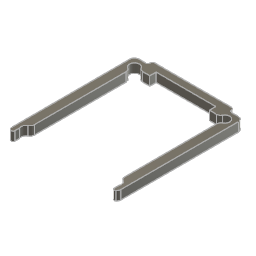
Assy v13 (Autodesk Fusion 360 archive; units mm, degrees)
design "Screen Spacer"
Autodesk Fusion 360 part; units mm, degrees
sketch "Sketch1" plane through (0, 0, 0) normal (0, 1, 0) x (1, 0, 0)
  line L0 (0, 0) -> (20, 0) construction
  line L1 (20, 0) -> (20, 24) construction
  line L2 (20, 24) -> (0, 24) construction
  line L3 (0, 24) -> (0, 0) construction
  circle A0 centre (0, 24) radius 1.1
  circle A1 centre (20, 24) radius 1.1
  circle A2 centre (20, 0) radius 1.1
  circle A3 centre (0, 0) radius 1.1
  line L4 (-2, 26) -> (22, 26)
  line L5 (22, 26) -> (22, -2)
  line L6 (22, -2) -> (-2, -2)
  line L7 (-2, -2) -> (-2, 26)
  line L8 (0, 24) -> (20, 24)
  line L9 (20, 24) -> (20, 0)
  line L10 (20, 0) -> (0, 0)
  line L11 (0, 0) -> (0, 24)
  dimension "d1" = 24
  dimension "d2" = 20
  dimension "d3" = 2.2
  dimension "d4" = 2
  dimension "d5" = 2
  dimension "d6" = 2
  dimension "d7" = 2
  constraint horizontal L0
  constraint vertical L1
  constraint horizontal L2
  constraint vertical L3
  constraint coincident L0.start L3.end
  constraint coincident L2.end L3.start
  constraint coincident L1.end L2.start
  constraint coincident L0.end L1.start
  constraint equal A0 A3
  constraint equal A0 A1
  constraint equal A1 A2
  constraint horizontal L4
  constraint vertical L5
  constraint horizontal L6
  constraint vertical L7
  constraint horizontal L8
  constraint vertical L9
  constraint horizontal L10
  constraint vertical L11
  measures "d1" distance of L0.start L2.end
  measures "d2" distance of L1.end L2.end
  measures "d3" diameter of A0
  measures "d4" distance of L2 L4
  measures "d5" distance of L1 L5
  measures "d6" distance of L0 L6
  measures "d7" distance of L3 L7
extrude "Extrude1" add sketch "Sketch1" along normal blind 2
fillet "Fillet1" radius 1 8 edges at (1.1, 1, -24) (0, 1, -22.9) (0, 1, -1.1) (18.9, 1, -24) (1.1, 1, 0) (20, 1, -22.9) (20, 1, -1.1) (18.9, 1, 0)
fillet "Fillet2" radius 1 4 edges at (-2, 1, -26) (-2, 1, 2) (22, 1, 2) (22, 1, -26)
extrude "Extrude2" cut 1 faces at (13.6667, 0.6667, 2) along direction (0, 0, -1) up to surface (2 mm away)
fillet "Fillet3" radius 0.4 2 edges at (-1, 1, 2) (21, 1, 2)
sketch "Sketch2" plane through (0, 2, 0) normal (0, 1, 0) x (-1, 0, 0)
  arc A0 (-21, 1.4472) -> (-21.6667, 1.7454) centre (-21.4, 1.4472) ccw
  arc A1 (-21.6667, 1.7454) -> (-22, 1) centre (-21, 1) ccw
  line L0 (-22, 1) -> (-22, -25)
  arc A2 (-22, -25) -> (-21, -26) centre (-21, -25) ccw
  line L1 (-21, -26) -> (1, -26)
  arc A3 (1, -26) -> (2, -25) centre (1, -25) ccw
  line L2 (2, -25) -> (2, 1)
  arc A4 (2, 1) -> (1.6667, 1.7454) centre (1, 1) ccw
  arc A5 (1.6667, 1.7454) -> (1, 1.4472) centre (1.4, 1.4472) ccw
  line L3 (1, 1.4472) -> (1, 0.4583)
  arc A6 (0.5238, -0.9673) -> (1, 0.4583) centre (0, 0) ccw
  arc A7 (0.5238, -0.9673) -> (0, -1.8466) centre (1, -1.8466) ccw
  line L4 (0, -1.8466) -> (0, -22.1534)
  arc A8 (0, -22.1534) -> (0.5238, -23.0327) centre (1, -22.1534) ccw
  arc A9 (-0.9673, -24.5238) -> (0.5238, -23.0327) centre (0, -24) ccw
  arc A10 (-0.9673, -24.5238) -> (-1.8466, -24) centre (-1.8466, -25) ccw
  line L5 (-1.8466, -24) -> (-18.1534, -24)
  arc A11 (-18.1534, -24) -> (-19.0327, -24.5238) centre (-18.1534, -25) ccw
  arc A12 (-20.5238, -23.0327) -> (-19.0327, -24.5238) centre (-20, -24) ccw
  arc A13 (-20.5238, -23.0327) -> (-20, -22.1534) centre (-21, -22.1534) ccw
  line L6 (-20, -22.1534) -> (-20, -1.8466)
  arc A14 (-20, -1.8466) -> (-20.5238, -0.9673) centre (-21, -1.8466) ccw
  arc A15 (-21, 0.4583) -> (-20.5238, -0.9673) centre (-20, 0) ccw
  line L7 (-21, 0.4583) -> (-21, 1.4472)
  line L8 (-3.4, -24) -> (-16.6, -24)
  line L9 (-16.6, -24) -> (-16.6, -25.4)
  line L10 (-16.6, -25.4) -> (-3.4, -25.4)
  line L11 (-3.4, -25.4) -> (-3.4, -24)
  line L12 (-1, -26) -> (-1, -27)
  line L13 (-1, -27) -> (-19, -27)
  line L14 (-19, -27) -> (-19, -26)
  line L15 (-1, -26) -> (-19, -26)
  dimension "d18" = 1.4
  dimension "d19" = 13.2
  dimension "d20" = 1
  dimension "d21" = 18
  constraint horizontal L8
  constraint vertical L9
  constraint horizontal L10
  constraint vertical L11
  constraint coincident L5 L8.start
  constraint midpoint L5 L8
  constraint coincident L1 L12.start
  constraint perpendicular L1 L12
  constraint perpendicular L12 L13
  constraint coincident L1 L14.end
  constraint perpendicular L1 L14
  constraint midpoint L1 L15
  measures "d18" distance of L8.end L9.end
  measures "d19" distance of L9.end L10.end
  measures "d20" distance of L12.start L12.end
  measures "d21" distance of L12.end L13.end
extrude "Extrude3" cut sketch "Sketch2" against normal up to surface (2 mm away) contours L5 L8 L9 L10 L11
extrude "Extrude4" add sketch "Sketch2" against normal up to surface (2 mm away) contours L1 L12 L13 L14 L15
fillet "Fillet5" radius 0.5 4 edges at (1, 1, -26) (1, 1, -27) (19, 1, -27) (19, 1, -26)

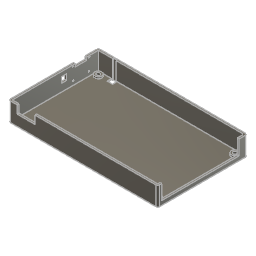
design "Main Case"
Autodesk Fusion 360 part; units mm, degrees
sketch "Sketch1" plane through (0, 0, 0) normal (0, 1, 0) x (1, 0, 0)
  line L0 (0, 0) -> (162, 0) construction
  line L1 (162, 0) -> (162, 95) construction
  line L2 (162, 95) -> (0, 95) construction
  line L3 (0, 95) -> (0, 0) construction
  line L4 (4, 91) -> (158, 91) construction
  line L5 (158, 91) -> (158, 4) construction
  line L6 (158, 4) -> (4, 4) construction
  line L7 (4, 4) -> (4, 91) construction
  circle A0 centre (4, 91) radius 2
  circle A1 centre (4, 4) radius 2
  circle A2 centre (158, 4) radius 2
  circle A3 centre (158, 91) radius 2
  line L8 (-1, 96) -> (163, 96)
  line L9 (163, 96) -> (163, -1)
  line L10 (163, -1) -> (-1, -1)
  line L11 (-1, -1) -> (-1, 96)
  line L12 (4, 91) -> (158, 4) construction
  line L13 (162, 95) -> (0, 0) construction
  dimension "d1" = 162
  dimension "d2" = 95
  dimension "d7" = 4
  dimension "d8" = 1
  dimension "d9" = 1
  dimension "d10" = 1
  dimension "d11" = 1
  dimension "d35" = 87
  dimension "d36" = 154
  constraint horizontal L0
  constraint vertical L1
  constraint horizontal L2
  constraint vertical L3
  constraint coincident L0.start L3.end
  constraint horizontal L4
  constraint vertical L5
  constraint horizontal L6
  constraint vertical L7
  constraint coincident L4.start L7.end
  constraint coincident L6.end L7.start
  constraint coincident L5.end L6.start
  constraint coincident L4.end L5.start
  constraint equal A0 A1
  constraint equal A1 A2
  constraint equal A2 A3
  constraint horizontal L8
  constraint vertical L9
  constraint horizontal L10
  constraint vertical L11
  constraint midpoint L12 L13
  measures "d1" distance of L1.end L2.end
  measures "d2" distance of L0.start L2.end
  measures "d7" diameter of A0
  measures "d8" distance of L2 L8
  measures "d9" distance of L1 L9
  measures "d10" distance of L0 L10
  measures "d11" distance of L3 L11
  measures "d35" distance of L4.start L6.end
  measures "d36" distance of L4.start L4.end
extrude "Extrude1" add sketch "Sketch1" along normal blind 1.2
sketch "Sketch2" plane through (0, 1.2, 0) normal (0, 1, 0) x (-1, 0, 0)
  circle A0 centre (-4, -91) radius 2
  circle A1 centre (-158, -4) radius 2
  circle A2 centre (-4, -4) radius 2
  circle A3 centre (-158, -91) radius 2
  line L0 (1, 1) -> (-163, 1)
  line L1 (-163, 1) -> (-163, -96)
  line L2 (-163, -96) -> (1, -96)
  line L3 (1, -96) -> (1, 1)
  circle A4 centre (-4, -91) radius 4
  circle A5 centre (-158, -91) radius 4
  circle A6 centre (-158, -4) radius 4
  circle A7 centre (-4, -4) radius 4
  dimension "d23" = 8
  constraint concentric A0 A4
  constraint concentric A3 A5
  constraint concentric A1 A6
  constraint concentric A2 A7
  constraint equal A4 A7
  constraint equal A4 A5
  constraint equal A5 A6
  measures "d23" diameter of A4
extrude "Extrude2" add sketch "Sketch2" along normal blind 2 contours A4 | A5 | A6 | A7
sketch "Sketch3" plane through (0, 0, 0) normal (0, -1, 0) x (1, 0, 0)
  circle A0 centre (4, -91) radius 2
  circle A1 centre (158, -4) radius 2
  circle A2 centre (4, -4) radius 2
  circle A3 centre (158, -91) radius 2
  line L0 (163, 1) -> (-1, 1)
  line L1 (-1, 1) -> (-1, -96)
  line L2 (-1, -96) -> (163, -96)
  line L3 (163, -96) -> (163, 1)
  line L4 (-1, 1) -> (163, 1)
  line L5 (163, 1) -> (163, -96)
  line L6 (163, -96) -> (-1, -96)
  line L7 (-1, -96) -> (-1, 1)
  line L8 (-3, 3) -> (165, 3)
  line L9 (165, 3) -> (165, -98)
  line L10 (165, -98) -> (-3, -98)
  line L11 (-3, -98) -> (-3, 3)
  dimension "d17" = 2
  dimension "d18" = 2
  dimension "d19" = 2
  dimension "d20" = 2
  constraint horizontal L4
  constraint vertical L5
  constraint horizontal L6
  constraint vertical L7
  constraint coincident L2.end L3.start
  constraint coincident L0.end L1.start
  constraint horizontal L8
  constraint vertical L9
  constraint horizontal L10
  constraint vertical L11
  measures "d17" distance of L4 L8
  measures "d18" distance of L7 L11
  measures "d19" distance of L6 L10
  measures "d20" distance of L5 L9
extrude "Extrude3" add sketch "Sketch3" against normal blind 21.3 contours L8 L9 L10 L11
fillet "Fillet1" radius 2 4 edges at (-3, 10.65, -98) (-3, 10.65, 3) (165, 10.65, 3) (165, 10.65, -98)
sketch "Sketch4" plane through (0, 1.2, 0) normal (0, 1, 0) x (-1, 0, 0)
  circle A0 centre (-4, -4) radius 4
  circle A1 centre (-4, -91) radius 4
  circle A2 centre (-158, -4) radius 4
  circle A3 centre (-158, -91) radius 4
  line L0 (1, 1) -> (-163, 1)
  line L1 (-163, 1) -> (-163, -96)
  line L2 (-163, -96) -> (1, -96)
  line L3 (1, -96) -> (1, 1)
  line L4 (-14, -96) -> (-20, -96)
  line L5 (-20, -96) -> (-20, -91)
  line L6 (-20, -91) -> (-14, -91)
  line L7 (-14, -91) -> (-14, -96)
  dimension "d30" = 6
  dimension "d31" = 5
  dimension "d32" = 15
  constraint horizontal L4
  constraint vertical L5
  constraint horizontal L6
  constraint vertical L7
  constraint coincident L2 L4.end
  measures "d30" distance of L4.start L4.end
  measures "d31" distance of L4.end L5.end
  measures "d32" distance of L2.end L4.start
extrude "Extrude4" cut sketch "Sketch4" against normal up to surface (1.2 mm away) contours L2 L4 L5 L6 L7
sketch "Sketch5" plane through (0, 21.3, 0) normal (0, 1, 0) x (-1, 0, 0)
  arc A0 (-165, -96) -> (-163, -98) centre (-163, -96) ccw
  line L0 (-163, -98) -> (1, -98)
  arc A1 (1, -98) -> (3, -96) centre (1, -96) ccw
  line L1 (3, -96) -> (3, 1)
  arc A2 (3, 1) -> (1, 3) centre (1, 1) ccw
  line L2 (1, 3) -> (-163, 3)
  arc A3 (-163, 3) -> (-165, 1) centre (-163, 1) ccw
  line L3 (-165, 1) -> (-165, -96)
  line L4 (1, -96) -> (-163, -96)
  line L5 (-163, -96) -> (-163, 1)
  line L6 (-163, 1) -> (1, 1)
  line L7 (1, 1) -> (1, -96)
  line L8 (-15, -96) -> (-19, -96)
  line L9 (-19, -96) -> (-19, -96.8)
  line L10 (-19, -96.8) -> (-15, -96.8)
  line L11 (-15, -96.8) -> (-15, -96)
  point P0 (-14, -96)
  dimension "d37" = 4
  dimension "d38" = 1
  dimension "d39" = 0.8
  constraint horizontal L8
  constraint vertical L9
  constraint horizontal L10
  constraint vertical L11
  constraint coincident L4 L8.start
  measures "d37" distance of L9.end L10.end
  measures "d38" distance of L8.start P0
  measures "d39" distance of L8.end L9.end
extrude "Extrude5" cut sketch "Sketch5" against normal up to surface (21.3 mm away) contours L4 L8 L9 L10 L11
sketch "Sketch6" plane through (165, 0, 0) normal (1, 0, 0) x (0, 0, -1)
  line L0 (96, 0) -> (96, 21.3)
  line L1 (96, 21.3) -> (-1, 21.3)
  line L2 (-1, 21.3) -> (-1, 0)
  line L3 (-1, 0) -> (96, 0)
  line L4 (1.7, 21.3) -> (88.7, 21.3)
  line L5 (88.7, 21.3) -> (88.7, 4.8)
  line L6 (88.7, 4.8) -> (1.7, 4.8)
  line L7 (1.7, 4.8) -> (1.7, 21.3)
  dimension "d42" = 2.7
  dimension "d43" = 87
  dimension "d44" = 4.8
  constraint horizontal L4
  constraint vertical L5
  constraint horizontal L6
  constraint vertical L7
  constraint coincident L1 L4.end
  measures "d42" distance of L2 L7
  measures "d43" distance of L4.start L4.end
  measures "d44" distance of L3 L5.end
extrude "Extrude6" cut sketch "Sketch6" against normal up to surface (2 mm away) contours L1 L4 L5 L6 L7
sketch "Sketch7" plane through (-3, 0, 0) normal (-1, 0, 0) x (0, 0, 1)
  line L0 (1, 0) -> (1, 21.3)
  line L1 (1, 21.3) -> (-96, 21.3)
  line L2 (-96, 21.3) -> (-96, 0) construction
  line L3 (-96, 0) -> (1, 0)
  line L4 (-85.5, 20) -> (-67.5, 20) construction
  line L5 (-67.5, 20) -> (-67.5, 6) construction
  line L6 (-67.5, 6) -> (-85.5, 6) construction
  line L7 (-85.5, 6) -> (-85.5, 20) construction
  line L8 (-83, 21.3) -> (-70, 21.3) construction
  line L9 (-70, 21.3) -> (-70, 18.7) construction
  line L10 (-70, 18.7) -> (-83, 18.7) construction
  line L11 (-83, 18.7) -> (-83, 21.3) construction
  line L12 (-83, 21.3) -> (-70, 18.7) construction
  circle A0 centre (-85.5, 20) radius 0.9
  circle A1 centre (-85.5, 6) radius 0.9
  circle A2 centre (-67.5, 6) radius 0.9
  circle A3 centre (-67.5, 20) radius 0.9
  dimension "d47" = 14
  dimension "d48" = 18
  dimension "d51" = 13
  dimension "d52" = 2.6
  dimension "d53" = 26
  dimension "d54" = 1.8
  constraint horizontal L4
  constraint vertical L5
  constraint horizontal L6
  constraint vertical L7
  constraint horizontal L8
  constraint vertical L9
  constraint horizontal L10
  constraint vertical L11
  constraint midpoint L4 L12
  constraint coincident L1 L8.end
  constraint coincident L4.start L7.end
  constraint coincident L6.end L7.start
  constraint coincident L5.end L6.start
  constraint coincident L4.end L5.start
  constraint equal A2 A3
  constraint equal A1 A2
  constraint equal A0 A1
  measures "d47" distance of L4.end L5.end
  measures "d48" distance of L4.start L4.end
  measures "d51" distance of L8.start L8.end
  measures "d52" distance of L8.start L10.end
  measures "d53" distance of L1.end L8.end
  measures "d54" diameter of A0
extrude "Extrude7" cut sketch "Sketch7" against normal up to surface (2 mm away)
sketch "Sketch8" plane through (-3, 0, 0) normal (-1, 0, 0) x (0, 0, 1)
  circle A0 centre (-67.5, 6) radius 0.9
  circle A1 centre (-85.5, 6) radius 0.9
  line L0 (1, 0) -> (1, 21.3)
  line L1 (1, 21.3) -> (-96, 21.3)
  line L2 (-96, 21.3) -> (-96, 0)
  line L3 (-96, 0) -> (1, 0)
  line L4 (-83, 21.3) -> (-70, 21.3)
  line L5 (-70, 21.3) -> (-70, 18.1)
  line L6 (-70, 18.1) -> (-83, 18.1)
  line L7 (-83, 18.1) -> (-83, 21.3)
  point P0 (-83, 21.3)
  point P1 (-70, 21.3)
  dimension "d59" = 3.2
  constraint horizontal L4
  constraint vertical L5
  constraint horizontal L6
  constraint vertical L7
  constraint coincident P0 L4.start
  constraint coincident L5 P1
  measures "d59" distance of P0 L6.end
extrude "Extrude8" cut sketch "Sketch8" against normal up to surface (2 mm away) contours L1 L4 L5 L6 L7
sketch "Sketch9" plane through (-3, 0, 0) normal (-1, 0, 0) x (0, 0, 1)
  line L0 (-83, 18.1) -> (-83, 21.3)
  line L1 (-83, 21.3) -> (-96, 21.3)
  line L2 (-96, 21.3) -> (-96, 0)
  line L3 (-96, 0) -> (1, 0)
  line L4 (1, 0) -> (1, 21.3)
  line L5 (1, 21.3) -> (-70, 21.3)
  line L6 (-70, 21.3) -> (-70, 18.1)
  line L7 (-70, 18.1) -> (-83, 18.1)
  circle A0 centre (-67.5, 20) radius 0.9
  circle A1 centre (-67.5, 6) radius 0.9
  circle A2 centre (-85.5, 20) radius 0.9
  circle A3 centre (-85.5, 6) radius 0.9
  line L8 (-60.2, 16.2) -> (-54.8, 16.2)
  line L9 (-54.8, 16.2) -> (-54.8, 9.8)
  line L10 (-54.8, 9.8) -> (-60.2, 9.8)
  line L11 (-60.2, 9.8) -> (-60.2, 16.2)
  line L12 (-67.5, 20) -> (-67.5, 6) construction
  line L13 (-67.5, 6) -> (-57.5, 13) construction
  line L14 (-57.5, 13) -> (-67.5, 20) construction
  line L15 (-60.2, 16.2) -> (-54.8, 9.8) construction
  dimension "d60" = 6.4
  dimension "d61" = 5.4
  dimension "d62" = 10
  constraint horizontal L8
  constraint vertical L9
  constraint horizontal L10
  constraint vertical L11
  constraint coincident A0.centre L12.start
  constraint coincident A1.centre L12.end
  constraint equal L13 L14
  constraint midpoint L13.end L15
  measures "d60" distance of L8.end L9.end
  measures "d61" distance of L8.start L8.end
  measures "d62" distance of L12 L13.end
extrude "Extrude9" cut sketch "Sketch9" against normal up to surface (2 mm away) contours L8 L9 L10 L11
sketch "Sketch10" plane through (0, 0, 3) normal (0, 0, 1) x (1, 0, 0)
  line L0 (163, 0) -> (163, 21.3)
  line L1 (163, 21.3) -> (-1, 21.3)
  line L2 (-1, 21.3) -> (-1, 0)
  line L3 (-1, 0) -> (163, 0)
  line L4 (6.5, 22.2) -> (26.5, 22.2)
  line L5 (26.5, 22.2) -> (26.5, 12.2)
  line L6 (26.5, 12.2) -> (6.5, 12.2)
  line L7 (6.5, 12.2) -> (6.5, 22.2)
  line L8 (6.5, 22.2) -> (26.5, 12.2) construction
  point P0 (16.5, 17.2)
  dimension "d66" = 20
  dimension "d67" = 10
  dimension "d68" = 17.2
  dimension "d69" = 17.5
  constraint horizontal L4
  constraint vertical L5
  constraint horizontal L6
  constraint vertical L7
  constraint midpoint L8 P0
  measures "d66" distance of L4.start L4.end
  measures "d67" distance of L4.end L5.end
  measures "d68" vertical distance of L2.end P0
  measures "d69" horizontal distance of L1.end P0
extrude "Extrude10" cut sketch "Sketch10" against normal up to surface (2 mm away) contours L1 L5 L6 L7
equation "d21 = -20.00 mm - 1.3 mm"
equation "d42 = 1.7 mm + 1 mm"
equation "d44 = 3.2 mm + 1.6 mm"
equation "d68 = 1.6 mm + 15.6 mm"

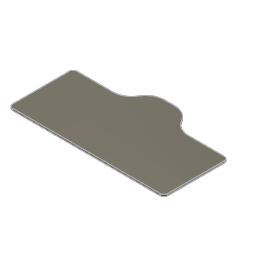
design "Culture Retainer Wall"
Autodesk Fusion 360 part; units mm, degrees
sketch "Sketch1" plane through (0, 0, 0) normal (0, 1, 0) x (1, 0, 0)
  line L0 (0, 0) -> (82, 0)
  line L1 (82, 0) -> (82, 34)
  line L2 (82, 34) -> (0, 34)
  line L3 (0, 34) -> (0, 0)
  line L4 (31, 44) -> (51, 44)
  line L5 (51, 44) -> (51, 34)
  line L6 (51, 34) -> (31, 34)
  line L7 (31, 34) -> (31, 44)
  dimension "d1" = 82
  dimension "d2" = 34
  dimension "d3" = 20
  dimension "d4" = 10
  constraint horizontal L0
  constraint vertical L1
  constraint horizontal L2
  constraint vertical L3
  constraint coincident L0.start L3.end
  constraint horizontal L4
  constraint vertical L5
  constraint horizontal L6
  constraint vertical L7
  constraint midpoint L2 L6
  measures "d1" distance of L1.end L2.end
  measures "d2" distance of L0.start L2.end
  measures "d3" distance of L4.start L4.end
  measures "d4" distance of L4.end L5.end
extrude "Extrude1" add sketch "Sketch1" along normal blind 1
fillet "Fillet1" radius 10 4 edges at (51, 0.5, -34) (51, 0.5, -44) (31, 0.5, -44) (31, 0.5, -34)
fillet "Fillet2" radius 2 4 edges at (0, 0.5, 0) (82, 0.5, 0) (82, 0.5, -34) (0, 0.5, -34)

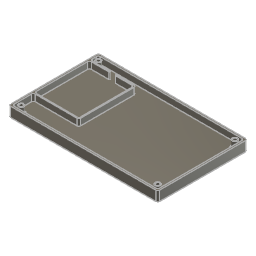
design "Bottom Case (Battery Tray)"
Autodesk Fusion 360 part; units mm, degrees
sketch "Sketch1" plane through (0, 0, 0) normal (0, 1, 0) x (1, 0, 0)
  line L0 (0, 0) -> (162, 0) construction
  line L1 (162, 0) -> (162, 95) construction
  line L2 (162, 95) -> (0, 95) construction
  line L3 (0, 95) -> (0, 0) construction
  line L4 (4, 91) -> (158, 91) construction
  line L5 (158, 91) -> (158, 4) construction
  line L6 (158, 4) -> (4, 4) construction
  line L7 (4, 4) -> (4, 91) construction
  circle A0 centre (4, 91) radius 2
  circle A1 centre (4, 4) radius 2
  circle A2 centre (158, 4) radius 2
  circle A3 centre (158, 91) radius 2
  line L8 (-1, 96) -> (163, 96)
  line L9 (163, 96) -> (163, -1)
  line L10 (163, -1) -> (-1, -1)
  line L11 (-1, -1) -> (-1, 96)
  line L12 (4, 91) -> (158, 4) construction
  line L13 (162, 95) -> (0, 0) construction
  dimension "d1" = 162
  dimension "d2" = 95
  dimension "d7" = 4
  dimension "d8" = 1
  dimension "d9" = 1
  dimension "d10" = 1
  dimension "d11" = 1
  dimension "d55" = 87
  dimension "d56" = 154
  constraint horizontal L0
  constraint vertical L1
  constraint horizontal L2
  constraint vertical L3
  constraint coincident L0.start L3.end
  constraint horizontal L4
  constraint vertical L5
  constraint horizontal L6
  constraint vertical L7
  constraint coincident L4.start L7.end
  constraint coincident L6.end L7.start
  constraint coincident L5.end L6.start
  constraint coincident L4.end L5.start
  constraint equal A0 A1
  constraint equal A1 A2
  constraint equal A2 A3
  constraint horizontal L8
  constraint vertical L9
  constraint horizontal L10
  constraint vertical L11
  constraint midpoint L12 L13
  measures "d1" distance of L1.end L2.end
  measures "d2" distance of L0.start L2.end
  measures "d7" diameter of A0
  measures "d8" distance of L2 L8
  measures "d9" distance of L3 L11
  measures "d10" distance of L0 L10
  measures "d11" distance of L1 L9
  measures "d55" distance of L4.start L6.end
  measures "d56" distance of L4.start L4.end
extrude "Extrude1" add sketch "Sketch1" along normal blind 3
sketch "Sketch2" plane through (0, 0, 0) normal (0, -1, 0) x (1, 0, 0)
  circle A0 centre (4, -91) radius 2
  circle A1 centre (158, -4) radius 2
  circle A2 centre (4, -4) radius 2
  circle A3 centre (158, -91) radius 2
  line L0 (163, 1) -> (-1, 1)
  line L1 (-1, 1) -> (-1, -96)
  line L2 (-1, -96) -> (163, -96)
  line L3 (163, -96) -> (163, 1)
  line L4 (-3, 3) -> (165, 3)
  line L5 (165, 3) -> (165, -98)
  line L6 (165, -98) -> (-3, -98)
  line L7 (-3, -98) -> (-3, 3)
  dimension "d16" = 2
  dimension "d17" = 2
  dimension "d18" = 2
  dimension "d19" = 2
  constraint horizontal L4
  constraint vertical L5
  constraint horizontal L6
  constraint vertical L7
  measures "d16" distance of L0 L4
  measures "d17" distance of L2 L6
  measures "d18" distance of L1 L7
  measures "d19" distance of L3 L5
extrude "Extrude2" add sketch "Sketch2" against normal blind 9 contours L4 L5 L6 L7
fillet "Fillet2" radius 2 4 edges at (-3, 4.5, 3) (-3, 4.5, -98) (165, 4.5, -98) (165, 4.5, 3)
sketch "Sketch3" plane through (0, 3, 0) normal (0, 1, 0) x (-1, 0, 0)
  circle A0 centre (-4, -91) radius 2
  circle A1 centre (-158, -4) radius 2
  circle A2 centre (-4, -4) radius 2
  circle A3 centre (-158, -91) radius 2
  line L0 (1, 1) -> (-163, 1)
  line L1 (-163, 1) -> (-163, -96)
  line L2 (-163, -96) -> (1, -96)
  line L3 (1, -96) -> (1, 1)
  line L4 (1, -86) -> (-49, -86)
  line L5 (-49, -86) -> (-49, -24)
  line L6 (-49, -24) -> (1, -24)
  line L7 (1, -24) -> (1, -86)
  line L8 (1, -87.2) -> (-50.2, -87.2)
  line L9 (-50.2, -87.2) -> (-50.2, -22.8)
  line L10 (-50.2, -22.8) -> (1, -22.8)
  point P0 (-24, -86)
  dimension "d24" = 50
  dimension "d25" = 62
  dimension "d26" = 10
  dimension "d28" = 1.2
  dimension "d29" = 1.2
  dimension "d30" = 1.2
  constraint horizontal L4
  constraint vertical L5
  constraint horizontal L6
  constraint vertical L7
  constraint midpoint L4 P0
  constraint coincident L3 L4.start
  constraint coincident L3 L8.start
  constraint perpendicular L3 L8
  constraint perpendicular L8 L9
  constraint coincident L3 L10.end
  constraint perpendicular L3 L10
  measures "d24" distance of L4.start L4.end
  measures "d25" distance of L4.end L5.end
  measures "d26" distance of L2 L4
  measures "d28" distance of L4 L8
  measures "d29" distance of L5 L9
  measures "d30" distance of L6 L10
extrude "Extrude3" add sketch "Sketch3" along normal up to surface (6 mm away) contours L3 L4 L5 L6 L8 L9 L10
fillet "Fillet3" radius 2 4 edges at (-1, 6, -22.8) (50.2, 6, -22.8) (50.2, 6, -87.2) (-1, 6, -87.2)
sketch "Sketch4" plane through (0, 9, 0) normal (0, 1, 0) x (-1, 0, 0)
  arc A0 (-50.2, -85.2) -> (-48.2, -87.2) centre (-48.2, -85.2) ccw
  line L0 (-48.2, -87.2) -> (-1, -87.2)
  arc A1 (1, -89.2) -> (-1, -87.2) centre (-1, -89.2) ccw
  line L1 (1, -89.2) -> (1, -96)
  line L2 (1, -96) -> (-163, -96)
  line L3 (-163, -96) -> (-163, 1)
  line L4 (-163, 1) -> (1, 1)
  line L5 (1, 1) -> (1, -20.8)
  arc A2 (-1, -22.8) -> (1, -20.8) centre (-1, -20.8) ccw
  line L6 (-1, -22.8) -> (-48.2, -22.8)
  arc A3 (-48.2, -22.8) -> (-50.2, -24.8) centre (-48.2, -24.8) ccw
  line L7 (-50.2, -24.8) -> (-50.2, -85.2)
  arc A4 (-163, 3) -> (-165, 1) centre (-163, 1) ccw
  line L8 (-165, 1) -> (-165, -96)
  arc A5 (-165, -96) -> (-163, -98) centre (-163, -96) ccw
  line L9 (-163, -98) -> (1, -98)
  arc A6 (1, -98) -> (3, -96) centre (1, -96) ccw
  line L10 (3, -96) -> (3, 1)
  arc A7 (3, 1) -> (1, 3) centre (1, 1) ccw
  line L11 (1, 3) -> (-163, 3)
  line L12 (1, -86) -> (-49, -86)
  line L13 (-49, -86) -> (-49, -24)
  line L14 (-49, -24) -> (1, -24)
  line L15 (1, -24) -> (1, -86)
  line L16 (-21.6, -87.2) -> (-27.6, -87.2)
  line L17 (-27.6, -87.2) -> (-27.6, -86)
  line L18 (-27.6, -86) -> (-21.6, -86)
  line L19 (-21.6, -86) -> (-21.6, -87.2)
  point P0 (-162.5, 1)
  point P1 (-162.5, -96)
  point P2 (1, -96)
  point P3 (1, 1)
  point P4 (-162, 0)
  point P5 (-162, -95)
  point P6 (0, -95)
  dimension "d35" = 6
  constraint horizontal L16
  constraint vertical L17
  constraint horizontal L18
  constraint vertical L19
  constraint coincident L12 L17.end
  constraint coincident L0 L16.start
  constraint midpoint L0 L16
  measures "d35" distance of L16.start L16.end
extrude "Extrude4" cut sketch "Sketch4" against normal up to surface (6 mm away) contours L0 L12 L16 L17 L18 L19
fillet "Fillet4" radius 2 4 edges at (-1, 6, -86) (49, 6, -86) (49, 6, -24) (-1, 6, -24)
fillet "Fillet5" radius 2 4 edges at (-1, 6, -96) (163, 6, -96) (163, 6, 1) (-1, 6, 1)
fillet "Fillet6" radius 0.6 4 edges at (21.6, 6, -86) (21.6, 6, -87.2) (27.6, 6, -86) (27.6, 6, -87.2)
sketch "Sketch5" plane through (0, 3, 0) normal (0, 1, 0) x (-1, 0, 0)
  circle A0 centre (-4, -91) radius 2
  circle A1 centre (-158, -4) radius 2
  circle A2 centre (-4, -4) radius 2
  circle A3 centre (-158, -91) radius 2
  arc A4 (1, -1) -> (-1, 1) centre (-1, -1) ccw
  line L0 (-1, 1) -> (-161, 1)
  arc A5 (-161, 1) -> (-163, -1) centre (-161, -1) ccw
  line L1 (-163, -1) -> (-163, -94)
  arc A6 (-163, -94) -> (-161, -96) centre (-161, -94) ccw
  line L2 (-161, -96) -> (-1, -96)
  arc A7 (-1, -96) -> (1, -94) centre (-1, -94) ccw
  line L3 (1, -94) -> (1, -89.2)
  arc A8 (1, -89.2) -> (-1, -87.2) centre (-1, -89.2) ccw
  line L4 (-1, -87.2) -> (-21, -87.2)
  arc A9 (-21, -86) -> (-21, -87.2) centre (-21, -86.6) ccw
  line L5 (-21, -86) -> (-1, -86)
  arc A10 (-1, -86) -> (1, -84) centre (-1, -84) ccw
  line L6 (1, -84) -> (1, -26)
  arc A11 (1, -26) -> (-1, -24) centre (-1, -26) ccw
  line L7 (-1, -24) -> (-47, -24)
  arc A12 (-47, -24) -> (-49, -26) centre (-47, -26) ccw
  line L8 (-49, -26) -> (-49, -84)
  arc A13 (-49, -84) -> (-47, -86) centre (-47, -84) ccw
  line L9 (-47, -86) -> (-28.2, -86)
  arc A14 (-28.2, -87.2) -> (-28.2, -86) centre (-28.2, -86.6) ccw
  line L10 (-28.2, -87.2) -> (-48.2, -87.2)
  arc A15 (-50.2, -85.2) -> (-48.2, -87.2) centre (-48.2, -85.2) ccw
  line L11 (-50.2, -85.2) -> (-50.2, -24.8)
  arc A16 (-48.2, -22.8) -> (-50.2, -24.8) centre (-48.2, -24.8) ccw
  line L12 (-48.2, -22.8) -> (-1, -22.8)
  arc A17 (-1, -22.8) -> (1, -20.8) centre (-1, -20.8) ccw
  line L13 (1, -20.8) -> (1, -1)
  circle A18 centre (-4, -91) radius 3
  circle A19 centre (-158, -91) radius 3
  circle A20 centre (-158, -4) radius 3
  circle A21 centre (-4, -4) radius 3
  dimension "d44" = 6
  constraint concentric A0 A18
  constraint concentric A3 A19
  constraint concentric A1 A20
  constraint concentric A2 A21
  constraint equal A18 A21
  constraint equal A18 A19
  constraint equal A19 A20
  measures "d44" diameter of A18
extrude "Extrude5" add sketch "Sketch5" along normal up to surface (7.5 mm away) contours A18 | A19 | A20 | A21
fillet "Fillet7" radius 1 4 edges at (6.797, 3, -2.9152) (6.797, 3, -89.9152) (160.797, 3, -89.9152) (160.797, 3, -2.9152)
extrude "Extrude6" add 1 faces at (106.0424, 0, -61.6396) along direction (0, -1, 0) blind 0.6
sketch "Sketch6" plane through (0, -0.6, 0) normal (0, -1, 0) x (1, 0, 0)
  arc A0 (165, 1) -> (163, 3) centre (163, 1) ccw
  line L0 (163, 3) -> (-1, 3)
  arc A1 (-1, 3) -> (-3, 1) centre (-1, 1) ccw
  line L1 (-3, 1) -> (-3, -96)
  arc A2 (-3, -96) -> (-1, -98) centre (-1, -96) ccw
  line L2 (-1, -98) -> (163, -98)
  arc A3 (163, -98) -> (165, -96) centre (163, -96) ccw
  line L3 (165, -96) -> (165, 1)
  circle A4 centre (4, -91) radius 2
  circle A5 centre (158, -4) radius 2
  circle A6 centre (4, -4) radius 2
  circle A7 centre (158, -91) radius 2
  circle A8 centre (4, -4) radius 4
  circle A9 centre (158, -4) radius 4
  circle A10 centre (158, -91) radius 4
  circle A11 centre (4, -91) radius 4
  dimension "d51" = 8
  constraint concentric A6 A8
  constraint concentric A5 A9
  constraint concentric A7 A10
  constraint concentric A4 A11
  constraint equal A8 A9
  constraint equal A9 A10
  constraint equal A10 A11
  measures "d51" diameter of A8
extrude "Extrude7" cut sketch "Sketch6" against normal blind 3 contours A8 | A9 | A10 | A11
extrude "Extrude8" add 1 faces at (-2.3333, 9, -40.3333) along direction (0, 1, 0) blind 1.5

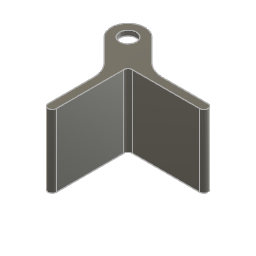
design "Culture Retainer"
Autodesk Fusion 360 part; units mm, degrees
sketch "Sketch1" plane through (0, 0, 0) normal (0, 1, 0) x (1, 0, 0)
  circle A0 centre (0, 0) radius 2
  line L0 (0, 0) -> (4.2, -4.2) construction
  line L1 (4.2, -4.2) -> (24.2, -4.2)
  line L2 (24.2, -4.2) -> (24.2, -6.2)
  line L3 (24.2, -6.2) -> (4.2, -6.2)
  line L4 (4.2, -6.2) -> (4.2, -4.2)
  line L5 (4.2, -4.2) -> (6.2, -4.2)
  line L6 (6.2, -4.2) -> (6.2, -24.2)
  line L7 (6.2, -24.2) -> (4.2, -24.2)
  line L8 (4.2, -24.2) -> (4.2, -4.2)
  line L9 (4.2, -9.8569) -> (-5.6569, 0)
  line L10 (-5.6569, 0) -> (0, 5.6569)
  line L11 (0, 5.6569) -> (9.8569, -4.2)
  line L12 (0, 0) -> (-2.8284, 2.8284)
  dimension "d1" = 4
  dimension "d2" = 4.2
  dimension "d3" = 4.2
  dimension "d4" = 2
  dimension "d5" = 20
  dimension "d6" = 135
  dimension "d7" = 4
  dimension "d8" = 8
  constraint coincident A0.centre L0.start
  constraint horizontal L1
  constraint vertical L2
  constraint horizontal L3
  constraint vertical L4
  constraint horizontal L5
  constraint vertical L6
  constraint horizontal L7
  constraint vertical L8
  constraint equal L2 L7
  constraint equal L1 L6
  constraint coincident L8 L9.start
  constraint perpendicular L9 L10
  constraint coincident L1 L11.end
  constraint perpendicular L10 L11
  constraint perpendicular L10 L12
  constraint midpoint L10 L12.end
  measures "d1" diameter of A0
  measures "d2" horizontal distance of A0.centre L0.end
  measures "d3" vertical distance of A0.centre L0.end
  measures "d4" distance of L1.end L2.end
  measures "d5" distance of L0.end L1.end
  measures "d6" angle of L1 L11
  measures "d7" distance of A0.centre L12.end
  measures "d8" distance of L9.end L10.end
extrude "Extrude1" add sketch "Sketch1" along normal blind 1.2
fillet "Fillet1" radius 1 5 edges at (6.2, 0.6, 6.2) (6.2, 0.6, 24.2) (4.2, 0.6, 24.2) (24.2, 0.6, 6.2) (24.2, 0.6, 4.2)
fillet "Fillet2" radius 4 2 edges at (-5.6569, 0.6, 0) (0, 0.6, -5.6569)
fillet "Fillet3" radius 6 2 edges at (4.2, 0.6, 9.8569) (9.8569, 0.6, 4.2)
sketch "Sketch2" plane through (0, 0, 0) normal (0, -1, 0) x (1, 0, 0)
  arc A0 (-2.8284, 2.8284) -> (2.8284, -2.8284) centre (0, 0) ccw
  line L0 (2.8284, -2.8284) -> (8.0995, 2.4426)
  arc A1 (12.3421, 4.2) -> (8.0995, 2.4426) centre (12.3421, -1.8) ccw
  line L1 (12.3421, 4.2) -> (23.2, 4.2)
  arc A2 (23.2, 4.2) -> (23.2, 6.2) centre (23.2, 5.2) ccw
  line L2 (23.2, 6.2) -> (7.2, 6.2)
  arc A3 (6.2, 7.2) -> (7.2, 6.2) centre (7.2, 7.2) ccw
  line L3 (6.2, 7.2) -> (6.2, 23.2)
  arc A4 (6.2, 23.2) -> (4.2, 23.2) centre (5.2, 23.2) ccw
  line L4 (4.2, 23.2) -> (4.2, 12.3421)
  arc A5 (2.4426, 8.0995) -> (4.2, 12.3421) centre (-1.8, 12.3421) ccw
  line L5 (2.4426, 8.0995) -> (-2.8284, 2.8284)
  circle A6 centre (0, 0) radius 2
  line L6 (4.2, 23.2) -> (4.2, 4.2)
  line L7 (4.2, 4.2) -> (23.2, 4.2)
  constraint coincident A4.end L4.start
  constraint coincident L1.end A2.start
  constraint perpendicular L6 L7
  constraint equal L6 L7
extrude "Extrude2" add sketch "Sketch2" along normal blind 16 contours L1 A2 L2 A3 L3 A4 L4 L6 L7
fillet "Fillet4" radius 2 1 edges at (4.2, -8, 4.2)
equation "d6 = 180 deg - 45 deg"
